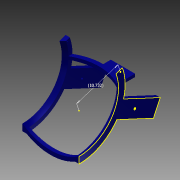
# Autodesk Inventor part: Inner
Saved by Autodesk Inventor 2014 (Build 180170000, 170)
## iProperties
Created: 2014-01-05
Part Number: Inner
Material: Polystyrene
Document SubType Name: Modeling
Designer: Tristan Debrunner
Density: 1.021 g/cm^3
Appearance: Smooth - White
Mass: 2714.34 g
Surface Area: 3377.29 cm^2
Volume: 2658.52 cm^3
Author: Tristan Debrunner
Autodesk Inventor part; units mm, degrees
ref_plane "YZ Plane" through (0, 0, 0) normal (1, 0, 0) x (0, 1, 0)
ref_plane "XY Plane" through (0, 0, 0) normal (0, 0, 1) x (1, 0, 0)
sketch "Sketch1" plane through (0, 0, 0) normal (0, 0, 1) x (1, 0, 0)
  line L0 (0, 0) -> (0, -41.796)
  line L1 (25.4, -16.396) -> (25.4, -41.796)
  arc A0 (0, 0) -> (25.4, -16.396) centre (177.8, 247.5686) ccw
  line L2 (355.6, 0) -> (355.6, -41.796)
  line L3 (330.2, -16.396) -> (330.2, -41.796)
  arc A1 (330.2, -16.396) -> (355.6, 0) centre (177.8, 247.5686) ccw
  line L4 (177.8, 247.5686) -> (533.4, 247.5686)
  line L5 (25.4, -41.796) -> (0, -41.796)
  line L6 (330.2, -41.796) -> (331.8938, -41.796)
  line L7 (331.8938, -41.796) -> (355.6, -41.796)
  constraints: 16 end point, 4 point on circle, 2 centre point, 2 parallel, 2 vertical
revolve "Revolution1" add sketch "Sketch1" angle 110 about axis through (177.8, 247.5686, 0) along (1, 0, 0)
sketch "Sketch2" plane through (0, -41.796, 0) normal (0, 0, 1) x (1, 0, 0)
  line L0 (25.4, 0) -> (25.4, 25.4) projected
  line L1 (355.6, 41.796) -> (355.6, 0) projected
  arc A0 (330.2, 25.4) -> (355.6, 41.796) centre (177.8, 289.3645) ccw projected
  line L2 (330.2, 0) -> (330.2, 25.4) projected
  arc A1 (25.4, 25.4) -> (330.2, 25.4) centre (177.8, 289.3645) ccw
  arc A2 (25.4, 0) -> (330.2, 0) centre (177.8, 263.9645) ccw
  line L3 (25.4, 25.4) -> (25.4, 0)
  line L4 (330.2, 25.4) -> (330.2, 0)
  line L5 (177.8, 289.3645) -> (533.4, 289.3645)
  line L6 (355.6, 0) -> (330.2, 0) projected
  dimension "d6" = 304.8
  dimension "d7" = 304.8
  constraints: 6 end point, 4 point on circle, 2 centre point, 2 equal length
  measures "d6" radius of A1
  measures "d7" radius of A2
revolve "Revolution2" add sketch "Sketch2" angle 4 about axis through (177.8, 247.5686, 0) along (1, 0, 0) contours L0 A1 L2 A2
ref_plane "Work Plane1" through (0, 304.8, 0) normal (0, 1, 0) x (-1, 0, 0)
ref_plane "Work Plane2" through (533.4, 247.5686, 0) normal (0, 1, 0) x (-1, 0, 0)
sketch "Sketch8" plane through (533.4, 247.5686, 0) normal (0, 1, 0) x (-1, 0, 0)
  arc A0 (177.8, -247.5686) -> (203.2, -263.9645) centre (355.6, 0) ccw projected
  line L0 (203.2, -263.9645) -> (203.2, -289.3645) projected
  line L1 (203.2, -289.3645) -> (177.8, -289.3645) projected
  line L2 (177.8, -289.3645) -> (177.8, -247.5686) projected
  line L3 (508, -289.3645) -> (508, -263.9645) projected
  line L4 (533.4, -247.5686) -> (533.4, -289.3645) projected
  line L5 (533.4, -289.3645) -> (508, -289.3645) projected
  arc A1 (203.2, -263.9645) -> (508, -263.9645) centre (355.6, 0) ccw
  arc A2 (203.2, -289.3645) -> (508, -289.3645) centre (355.6, -25.4) ccw
  line L6 (203.2, -289.3645) -> (203.2, -263.9645)
  line L7 (508, -263.9645) -> (508, -289.3645)
  line L8 (355.6, 0) -> (533.4, 0)
  arc A3 (508, -263.9645) -> (533.4, -247.5686) centre (355.6, 0) ccw projected
  dimension "d44" = 304.8
  dimension "d45" = 304.8
  constraints: 6 end point, 4 point on circle, 2 centre point, 1 parallel, 1 perpendicular
  measures "d44" radius of A1
  measures "d45" radius of A2
revolve "Revolution4" add sketch "Sketch8" angle 4 about axis through (177.8, 247.5686, 0) along (-1, 0, 0) contours A1 L3 A2 L0
sketch "Sketch9" plane through (25.4, 247.5686, -263.9645) normal (1, 0, 0) x (0, 0, -1)
  line L0 (0, 0) -> (25.4, 0) projected
  line L1 (-15.919, 90.2812) -> (7.9492, 98.9685) projected
  line L2 (-3.9849, 94.6248) -> (-3.9849, 81.9248)
  point P0 (-263.9645, -247.5686)
  dimension "d47" = 12.7
  constraints: 2 end point, 1 midpoint, 1 perpendicular
  measures "d47" distance of L2.start L2.end
hole "Hole3" at (25.4, 329.4934, -259.9796) direction (1, 0, 0) diameter 6.35 end through all
hole "Hole4" at (25.4, 329.4934, -259.9796) direction (-1, 0, 0) diameter 6.35 end through all
sketch "Sketch10" plane through (355.6, -41.796, 0) normal (1, 0, 0) x (0, 0, -1)
  arc A0 (0, 0) -> (271.9137, 388.333) centre (0, 289.3645) ccw projected
  line L0 (237.0336, 123.3919) -> (467.2357, 16.0468)
  line L1 (165.9727, 52.331) -> (419.9727, 52.331) construction
  line L2 (279.5047, 214.4715) -> (509.7069, 107.1264)
  line L3 (237.0336, 123.3919) -> (491.0336, 123.3919) construction
  line L4 (509.7069, 107.1264) -> (467.2357, 16.0468)
  arc A1 (237.0336, 123.3919) -> (279.5047, 214.4715) centre (0, 289.3645) ccw
  dimension "d65" = 254
  dimension "d66" = 25
  dimension "d67" = 254
  dimension "d68" = 25
  constraints: 10 end point, 2 equal length, 2 horizontal, 2 point on circle, 1 centre point, 1 concentric, 1 parallel, 1 perpendicular
  measures "d65" distance of L0.start L0.end
  measures "d66" angle of L0 L1
  measures "d67" distance of L2.start L2.end
  measures "d68" angle of L2 L3
extrude "Extrusion3" add sketch "Sketch10" against normal blind 25.4
sketch "Sketch11" plane through (0, -41.796, 0) normal (-1, 0, 0) x (0, 0, 1)
  arc A0 (-271.9137, 388.333) -> (0, 0) centre (0, 289.3645) ccw projected
  line L0 (-279.5047, 214.4715) -> (-509.7069, 107.1264) projected
  line L1 (-509.7069, 107.1264) -> (-467.2357, 16.0468) projected
  line L2 (-467.2357, 16.0468) -> (-237.0336, 123.3919) projected
extrude "Extrusion4" add sketch "Sketch11" against normal blind 25.4
sketch "Sketch12" plane through (0, -41.796, 0) normal (-1, 0, 0) x (0, 0, 1)
  line L0 (-509.7069, 107.1264) -> (-467.2357, 16.0468) projected
  line L1 (-467.2357, 16.0468) -> (-237.0336, 123.3919) projected
  line L2 (-488.4713, 61.5866) -> (-350.35, 125.9937)
  dimension "d73" = 152.4
  constraints: 2 end point, 1 midpoint, 1 parallel
  measures "d73" distance of L2.start L2.end
hole "Hole5" at (0, 84.1977, -350.35) direction (1, 0, 0) diameter 12.7 end through all
sketch "Sketch13" plane through (177.8, 247.5686, -25.4) normal (0, 1, 0) x (1, 0, 0)
  line L0 (152.4, 263.9645) -> (152.4, 238.5645) projected
  arc A0 (152.4, 238.5645) -> (-152.4, 238.5645) centre (0, -25.4) ccw projected
  line L1 (152.4, 263.9645) -> (152.4, 352.8645)
  line L2 (152.4, 352.8645) -> (76.2, 352.8645)
  line L3 (76.2, 279.4) -> (76.2, 269.7213)
  line L4 (119.5299, 269.7213) -> (119.5299, 257.7498)
  line L5 (119.5299, 257.7498) -> (152.4, 257.7498)
  line L6 (152.4, 263.9645) -> (152.4, 257.7498)
  line L7 (119.5299, 269.7213) -> (76.2, 269.7213)
  line L8 (-152.4, 238.5645) -> (-152.4, 263.9645) projected
  line L9 (76.2, 352.8645) -> (0, 352.8645)
  line L10 (0, 352.8645) -> (0, 279.4)
  line L11 (0, 279.4) -> (76.2, 279.4)
  point P0 (-177.8, -25.4)
  dimension "d81" = 88.9
  dimension "d82" = 76.2
  dimension "d85" = 76.2
  constraints: 20 end point, 7 perpendicular, 3 point on circle, 2 point on line, 1 parallel, 1 tangent
  measures "d81" distance of L0.start L1.end
  measures "d82" distance of L1.end L2.end
  measures "d85" distance of L2.end L9.end
extrude "Extrusion5" add sketch "Sketch13" against normal blind 18.288 contours L0 L5 L4 L7 L3 L11 L10 L9 L2 L1
sketch "Sketch14" plane through (355.6, -41.796, 0) normal (1, 0, 0) x (0, 0, -1)
  circle A0 centre (350.35, 125.9937) radius 6.35 projected
  circle A1 centre (259.9796, 371.2894) radius 3.175 projected
  line L0 (0, 41.796) -> (0, 0) projected
  arc A2 (0, 0) -> (237.0336, 123.3919) centre (0, 289.3645) ccw projected
  line L1 (237.0336, 123.3919) -> (467.2357, 16.0468) projected
  line L2 (467.2357, 16.0468) -> (509.7069, 107.1264) projected
  line L3 (509.7069, 107.1264) -> (279.5047, 214.4715) projected
  arc A3 (279.5047, 214.4715) -> (271.9137, 388.333) centre (0, 289.3645) ccw projected
  line L4 (232.6384, 374.038) -> (271.9137, 388.333) projected
  arc A4 (0, 41.796) -> (232.6384, 374.038) centre (0, 289.3645) ccw projected
  dimension "d86" = 272.5823
  measures "d86" distance of A1.centre A2.centre
body "Solid1"
